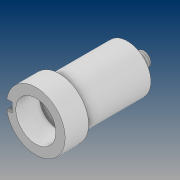
# Autodesk Inventor part: piraki
Saved by Autodesk Inventor 2021 (Build 250183000, 183)
## iProperties
Created: 2020-12-26
Part Number: piraki
Material: Generic
Document SubType Name: Modeling
Designer: Angelos
Density: 1 g/cm^3
Appearance: Default
Author: Angelos
Autodesk Inventor part; units mm, degrees
ref_plane "YZ Plane" through (0, 0, 0) normal (1, 0, 0) x (0, 1, 0)
ref_plane "XZ Plane" through (0, 0, 0) normal (0, 1, 0) x (-1, 0, 0)
ref_plane "XY Plane" through (0, 0, 0) normal (0, 0, 1) x (1, 0, 0)
sketch "Sketch1" plane through (0, 0, 0) normal (0, 0, 1) x (1, 0, 0)
  circle A0 centre (0, 0) radius 10
  circle A1 centre (0, 0) radius 12.5
  dimension "d0" = 0
  dimension "d1" = 0
  dimension "d2" = 0
  dimension "d3" = 0
  dimension "d4" = 25
  dimension "d5" = 20
  constraints: 2 centre point
  measures "d0" distance of point (0, 0) A1.centre
  measures "d1" distance of point (0, 0) A0.centre
  measures "d2" distance of point (0, 0) A0.centre
  measures "d3" distance of point (0, 0) A1.centre
  measures "d4" diameter of A1
  measures "d5" diameter of A0
extrude "Extrusion1" add sketch "Sketch1" along normal blind 10
extrude "Extrusion2" add sketch "Sketch1" against normal blind 29 contours A0
sketch "Sketch2" plane through (0, 0, -29) normal (0, 0, -1) x (-1, 0, 0)
  circle A0 centre (0, 0) radius 8.5
  dimension "d10" = 17
  constraints: 1 centre point, 1 coincident
  measures "d10" diameter of A0
extrude "Extrusion3" add sketch "Sketch2" along normal blind 1
sketch "Sketch3" plane through (0, 0, -30) normal (0, 0, -1) x (-1, 0, 0)
  circle A0 centre (0, 0) radius 3
  dimension "d13" = 6
  constraints: 1 centre point, 1 coincident
  measures "d13" diameter of A0
extrude "Extrusion4" add sketch "Sketch3" along normal blind 6
thread "Thread1" size "M6x1" class "6g" standard "ANSI Metric M Profile" full length
sketch "Sketch4" plane through (0, 0, 10) normal (0, 0, 1) x (1, 0, 0)
  circle A0 centre (0, 0) radius 10 projected
  line L0 (-10, 0) -> (-10, 2)
  line L1 (-10, 2) -> (-12.8956, 2)
  line L2 (-10, 0) -> (-11.1456, 0)
  line L3 (-10, 0) -> (-10, -2)
  line L4 (-10, -2) -> (-12.8956, -2)
  line L5 (-12.8956, -2) -> (-12.8956, 2)
  constraints: 12 end point, 3 vertical, 2 symmetric about line, 1 horizontal, 1 horizontal alignment, 1 perpendicular, 1 other
extrude "Extrusion5" cut sketch "Sketch4" against normal up to surface (10 mm away) contours L3 L4 L5 L1 L0
sketch "Sketch5" plane through (0, 0, 0) normal (0, 0, 1) x (1, 0, 0)
  circle A0 centre (0, 0) radius 10
  circle A1 centre (0, 0) radius 8.5
  point P0 (-10, 0)
  constraints: 2 coincident, 1 centre point, 1 horizontal alignment, 2 other
extrude "Extrusion6" add sketch "Sketch5" along normal blind 10
body "Solid1"
